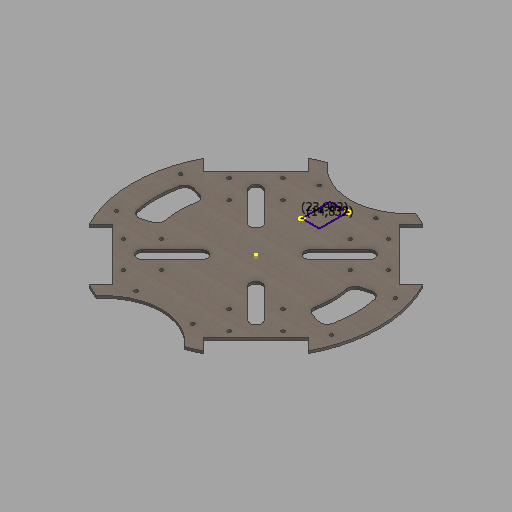
# Autodesk Inventor part: floor_v2
Saved by Autodesk Inventor 2023 (Build 270158000, 158)
## iProperties
Created: 2024-09-07
Part Number: floor_v2
Material: Алюминий 6061
Document SubType Name: Modeling
Designer: Ivan
Density: 2.7 g/cm^3
Appearance: Орех
Mass: 136.784 g
Surface Area: 534.847 cm^2
Volume: 50.6608 cm^3
Author: Ivan
Autodesk Inventor part; units mm, degrees
ref_plane "YZ Plane" through (0, 0, 0) normal (1, 0, 0) x (0, 1, 0)
ref_plane "XZ Plane" through (0, 0, 0) normal (0, 1, 0) x (-1, 0, 0)
ref_plane "XY Plane" through (0, 0, 0) normal (0, 0, 1) x (1, 0, 0)
sketch "Эскиз2" plane through (0, 0, 0) normal (0, 1, 0) x (1, 0, 0)
  circle A0 centre (0, 0) radius 107.5
  circle A1 centre (0, 0) radius 104
  line L0 (0, 0) -> (104, 0) construction
  line L1 (0, 0) -> (0, -104) construction
  line L2 (0, 0) -> (-104, 0) construction
  line L3 (0, 0) -> (0, 104) construction
  line L4 (104, 0) -> (0, -104) construction
  line L5 (0, 104) -> (-104, 0) construction
  line L6 (0, -104) -> (-104, 0) construction
  line L7 (104, 0) -> (0, 104) construction
  line L8 (0, 0) -> (-73.5391, -73.5391) construction
  line L9 (0, 0) -> (73.5391, -73.5391) construction
  line L10 (0, 0) -> (73.5391, 73.5391) construction
  line L11 (0, 0) -> (-73.5391, 73.5391) construction
  line L12 (-38.4471, -82.2877) -> (-82.2877, -38.4471)
  line L13 (-38.4471, -82.2877) -> (-48.2758, -92.1165)
  line L14 (-82.2877, -38.4471) -> (-92.1165, -48.2758)
  line L15 (92.1165, -48.2758) -> (82.2877, -38.4471)
  line L16 (82.2877, -38.4471) -> (38.4471, -82.2877)
  line L17 (38.4471, -82.2877) -> (48.2758, -92.1165)
  line L18 (48.2758, 92.1165) -> (38.4471, 82.2877)
  line L19 (38.4471, 82.2877) -> (82.2877, 38.4471)
  line L20 (82.2877, 38.4471) -> (92.1165, 48.2758)
  line L21 (-48.2758, 92.1165) -> (-38.4471, 82.2877)
  line L22 (-38.4471, 82.2877) -> (-82.2877, 38.4471)
  line L23 (-82.2877, 38.4471) -> (-92.1165, 48.2758)
  line L24 (0, -107.5) -> (0, -79.5) construction
  circle A2 centre (0, -116.5) radius 37 construction
  circle A3 centre (0, -127) radius 47.5
  line L25 (0, 107.5) -> (0, 79.5) construction
  circle A4 centre (0, 127) radius 47.5
  line L26 (-92.1165, 48.2758) -> (-94.7051, 50.8645)
  line L27 (-48.2758, 92.1165) -> (-50.8645, 94.7051)
  line L28 (48.2758, 92.1165) -> (50.8645, 94.7051)
  line L29 (92.1165, 48.2758) -> (94.7051, 50.8645)
  line L30 (92.1165, -48.2758) -> (94.7051, -50.8645)
  line L31 (48.2758, -92.1165) -> (50.8645, -94.7051)
  line L32 (-92.1165, -48.2758) -> (-94.7051, -50.8645)
  line L33 (-48.2758, -92.1165) -> (-50.8645, -94.7051)
  point P0 (-52, -52)
  point P1 (-52, 52)
  point P2 (52, 52)
  point P3 (52, -52)
  point P4 (-60.3674, -60.3674)
  point P5 (60.3674, -60.3674)
  point P6 (60.3674, 60.3674)
  point P7 (-60.3674, 60.3674)
  point P8 (-36.9892, -97.1998)
  point P9 (36.9892, -97.1998)
  point P10 (36.9892, 97.1998)
  point P11 (-36.9892, 97.1998)
  dimension "d137" = 215
  dimension "d138" = 208
  dimension "d143" = 74
  dimension "d144" = 95
  dimension "d140" = 62
  dimension "d141" = 13.9
  dimension "d142" = 28
  constraints: 68 end point, 15 point on line, 14 equal length, 10 perpendicular, 8 collinear, 8 midpoint, 5 parallel, 2 coincident, 2 horizontal, 2 vertical, 1 vertical alignment, 32 other
  measures "d140" distance from line of L14 L12.start
  measures "d141" distance from line of L12 L13.end
  measures "d142" distance of L24.start L24.end
extrude "Выдавливание1" add sketch "Эскиз2" along normal blind 2 contours A1 L15 L16 L17 A3 L13 L12 L14 L23 L22 L21 A4 L18 L19 L20
sketch "Эскиз3" plane through (0, 2, 0) normal (0, -1, 0) x (-1, 0, 0)
  line L0 (33.8509, 77.6915) -> (77.6915, 33.8509) construction
  line L1 (55.7712, 55.7712) -> (0, 0) construction
  line L2 (44.4575, 67.0849) -> (67.0849, 44.4575) construction
  circle A0 centre (44.4575, 67.0849) radius 1.5
  circle A1 centre (67.0849, 44.4575) radius 1.5
  line L3 (28.3991, 51.0265) -> (51.0265, 28.3991) construction
  circle A2 centre (28.3991, 51.0265) radius 1.5
  circle A3 centre (51.0265, 28.3991) radius 1.5
  line L4 (44.4575, -67.0849) -> (67.0849, -44.4575) construction
  line L5 (28.3991, -51.0265) -> (51.0265, -28.3991) construction
  line L6 (55.7712, -55.7712) -> (0, 0) construction
  line L7 (-44.4575, -67.0849) -> (-67.0849, -44.4575) construction
  line L8 (-28.3991, -51.0265) -> (-51.0265, -28.3991) construction
  line L9 (-55.7712, -55.7712) -> (0, 0) construction
  line L10 (-67.0849, 44.4575) -> (-44.4575, 67.0849) construction
  line L11 (-51.0265, 28.3991) -> (-28.3991, 51.0265) construction
  line L12 (-55.7712, 55.7712) -> (0, 0) construction
  circle A4 centre (-44.4575, 67.0849) radius 1.5
  circle A5 centre (-67.0849, 44.4575) radius 1.5
  circle A6 centre (-28.3991, 51.0265) radius 1.5
  circle A7 centre (-51.0265, 28.3991) radius 1.5
  circle A8 centre (-44.4575, -67.0849) radius 1.5
  circle A9 centre (-67.0849, -44.4575) radius 1.5
  circle A10 centre (-51.0265, -28.3991) radius 1.5
  circle A11 centre (-28.3991, -51.0265) radius 1.5
  circle A12 centre (44.4575, -67.0849) radius 1.5
  circle A13 centre (28.3991, -51.0265) radius 1.5
  circle A14 centre (51.0265, -28.3991) radius 1.5
  circle A15 centre (67.0849, -44.4575) radius 1.5
  line L13 (-38.4471, -82.2877) -> (-82.2877, -38.4471) projected
  line L14 (82.2877, -38.4471) -> (38.4471, -82.2877) projected
  line L15 (38.4471, 82.2877) -> (82.2877, 38.4471) projected
  line L16 (-82.2877, 38.4471) -> (-38.4471, 82.2877) projected
  line L17 (82.2877, 38.4471) -> (92.1165, 48.2758) projected
  point P0 (39.7128, 39.7128)
  point P1 (-39.7128, -39.7128)
  point P2 (39.7128, -39.7128)
  point P3 (-39.7128, 39.7128)
  point P4 (-40.1306, -40.1306)
  dimension "d83" = 16
  dimension "d84" = 3
  dimension "d85" = 3
  dimension "d86" = 22.71
  dimension "d87" = 3
  dimension "d88" = 3
  dimension "d89" = 22.71
  dimension "d90" = 22.71
  dimension "d91" = 22.71
  dimension "d95" = 3
  dimension "d96" = 3
  dimension "d97" = 3
  dimension "d98" = 3
  dimension "d99" = 3
  dimension "d100" = 3
  dimension "d101" = 3
  dimension "d102" = 3
  dimension "d103" = 3
  dimension "d104" = 3
  dimension "d105" = 3
  dimension "d106" = 3
  dimension "d145" = 6.5
  dimension "d146" = 6.5
  dimension "d147" = 6.5
  dimension "d148" = 6.5
  constraints: 26 end point, 16 centre point, 16 coincident, 10 point on line, 9 midpoint, 8 equal length, 8 parallel, 2 perpendicular, 1 collinear
  measures "d83" distance from line of L1 L2.start
  measures "d84" diameter of A0
  measures "d85" diameter of A1
  measures "d86" distance from line of L3 L1.start
  measures "d87" diameter of A2
  measures "d88" diameter of A3
  measures "d89" distance from line of L5 L6.start
  measures "d90" distance from line of L11 L12.start
  measures "d91" distance from line of L8 L9.start
  measures "d95" diameter of A4
  measures "d96" diameter of A5
  measures "d97" diameter of A6
  measures "d98" diameter of A7
  measures "d99" diameter of A8
  measures "d100" diameter of A9
  measures "d101" diameter of A10
  measures "d102" diameter of A11
  measures "d103" diameter of A12
  measures "d104" diameter of A13
  measures "d105" diameter of A14
  measures "d106" diameter of A15
  measures "d145" distance from line of L15 L1.start
  measures "d146" distance from line of L16 L12.start
  measures "d147" distance from line of L13 L9.start
  measures "d148" distance from line of L6.start L14
extrude "Выдавливание5" cut sketch "Эскиз3" along normal through all
sketch "Эскиз6" plane through (0, 2, 0) normal (0, -1, 0) x (-1, 0, 0)
  arc A0 (36.9892, -97.1998) -> (-36.9892, -97.1998) centre (0, -127) ccw projected
  arc A1 (-36.9892, 97.1998) -> (36.9892, 97.1998) centre (0, 127) ccw projected
  point P0 (-0.0301, 154.5629)
  point P1 (-0.0412, -154.5628)
sketch "Эскиз7" plane through (0, 2, 0) normal (0, -1, 0) x (-1, 0, 0)
  circle A0 centre (0, 0) radius 94.2655 construction
  circle A1 centre (-90.3481, 26.8924) radius 1.5
  circle A2 centre (-90.3481, -26.8924) radius 1.5
  circle A3 centre (90.3481, 26.8924) radius 1.5
  circle A4 centre (90.3481, -26.8924) radius 1.5
  line L0 (-92.1165, 48.2758) -> (-82.2877, 38.4471) projected
  line L1 (-82.2877, -38.4471) -> (-92.1165, -48.2758) projected
  line L2 (92.1165, -48.2758) -> (82.2877, -38.4471) projected
  line L3 (82.2877, 38.4471) -> (92.1165, 48.2758) projected
  dimension "d119" = 188.531
  dimension "d120" = 3
  dimension "d121" = 3
  dimension "d124" = 3
  dimension "d125" = 3
  dimension "d149" = 13.87
  dimension "d150" = 13.87
  dimension "d151" = 13.87
  dimension "d152" = 13.87
  constraints: 5 centre point, 4 point on circle, 1 coincident
  measures "d119" diameter of A0
  measures "d120" diameter of A1
  measures "d121" diameter of A2
  measures "d124" diameter of A3
  measures "d125" diameter of A4
  measures "d149" distance from line of L0 A1.centre
  measures "d150" distance from line of L1 A2.centre
  measures "d151" distance from line of L2 A4.centre
  measures "d152" distance from line of L3 A3.centre
extrude "Выдавливание4" cut sketch "Эскиз7" along normal through all
sketch "Эскиз8" plane through (0, 2, 0) normal (0, 1, 0) x (1, 0, 0)
  arc A0 (-48.2758, -92.1165) -> (-36.9892, -97.1998) centre (0, 0) ccw projected
  arc A1 (36.9892, -97.1998) -> (48.2758, -92.1165) centre (0, 0) ccw projected
  arc A2 (36.9892, -97.1998) -> (-36.9892, -97.1998) centre (0, -127) ccw projected
  circle A3 centre (0, -127) radius 55.4164 construction
  circle A4 centre (-23.8556, -76.9811) radius 1.5
  circle A5 centre (23.8556, -76.9811) radius 1.5
  circle A6 centre (-28.3991, -51.0265) radius 1.5 construction
  circle A7 centre (-51.0265, -28.3991) radius 1.5 construction
  circle A8 centre (-67.0849, -44.4575) radius 1.5 construction
  circle A9 centre (-44.4575, -67.0849) radius 1.5 construction
  circle A10 centre (-51.0265, -28.3991) radius 1.5 construction
  line L0 (-51.0265, -28.3991) -> (-28.3991, -51.0265) construction
  line L1 (-67.0849, -44.4575) -> (-44.4575, -67.0849) construction
  line L2 (-55.7712, -55.7712) -> (-39.7128, -39.7128) construction
  line L3 (-50.4184, -50.4184) -> (-23.8556, -76.9811) construction
  circle A11 centre (67.0849, -44.4575) radius 1.5 construction
  circle A12 centre (44.4575, -67.0849) radius 1.5 construction
  line L4 (44.4575, -67.0849) -> (67.0849, -44.4575) construction
  arc A13 (-92.1165, 48.2758) -> (-92.1165, -48.2758) centre (0, 0) ccw construction
  line L5 (-104, 0) -> (104, 0) construction
  arc A14 (92.1165, -48.2758) -> (92.1165, 48.2758) centre (0, 0) ccw construction
  circle A15 centre (-23.8556, 76.9811) radius 1.5
  circle A16 centre (23.8556, 76.9811) radius 1.5
  point P0 (-44.5136, -93.9922)
  point P1 (-104, 0)
  dimension "d153" = 11.2867
  dimension "d154" = 3.7622
  dimension "d156" = 22.71
  dimension "d157" = 7.57
  dimension "d158" = 7.57
  constraints: 12 end point, 7 point on circle, 5 centre point, 2 equal radius, 2 midpoint, 2 symmetric about line, 1 coincident, 1 horizontal, 1 perpendicular, 1 point on line, 2 other
  measures "d153" horizontal distance of A0.end A0.start
  measures "d154" horizontal distance of A3.start A0.start
  measures "d156" distance from line of L0 L2.start
  measures "d157" distance from line of L1 L3.start
  measures "d158" distance from line of L4 A5.centre
extrude "Выдавливание6" cut sketch "Эскиз8" against normal through all
sketch "Эскиз9" plane through (0, 2, 0) normal (0, 1, 0) x (1, 0, 0)
  circle A0 centre (-23.8556, 76.9811) radius 1.5 projected
  circle A1 centre (23.8556, -76.9811) radius 1.5 projected
  circle A2 centre (23.8556, 76.9811) radius 1.5 projected
  circle A3 centre (-23.8556, -76.9811) radius 1.5 projected
  circle A4 centre (-90.3481, 26.8924) radius 1.5 projected
  circle A5 centre (90.3481, -26.8924) radius 1.5 projected
  circle A6 centre (-90.3481, -26.8924) radius 1.5 projected
  circle A7 centre (90.3481, 26.8924) radius 1.5 projected
  circle A8 centre (51.0265, -28.3991) radius 1.5 projected
  circle A9 centre (-67.0849, -44.4575) radius 1.5 projected
  circle A10 centre (-44.4575, 67.0849) radius 1.5 projected
  circle A11 centre (51.0265, 28.3991) radius 1.5 projected
  circle A12 centre (28.3991, 51.0265) radius 1.5 projected
  circle A13 centre (-67.0849, 44.4575) radius 1.5 projected
  circle A14 centre (-28.3991, -51.0265) radius 1.5 projected
  circle A15 centre (28.3991, -51.0265) radius 1.5 projected
  circle A16 centre (67.0849, -44.4575) radius 1.5 projected
  circle A17 centre (-51.0265, -28.3991) radius 1.5 projected
  circle A18 centre (-28.3991, 51.0265) radius 1.5 projected
  circle A19 centre (67.0849, 44.4575) radius 1.5 projected
  circle A20 centre (44.4575, 67.0849) radius 1.5 projected
  circle A21 centre (-51.0265, 28.3991) radius 1.5 projected
  circle A22 centre (-44.4575, -67.0849) radius 1.5 projected
  circle A23 centre (44.4575, -67.0849) radius 1.5 projected
  line L0 (-82.2877, 38.4471) -> (-92.1165, 48.2758) projected
  arc A24 (-92.1165, 48.2758) -> (-92.1165, -48.2758) centre (0, 0) ccw projected
  line L1 (-92.1165, -48.2758) -> (-82.2877, -38.4471) projected
  line L2 (-82.2877, -38.4471) -> (-38.4471, -82.2877) projected
  line L3 (-38.4471, -82.2877) -> (-48.2758, -92.1165) projected
  arc A25 (-48.2758, -92.1165) -> (-36.9892, -97.1998) centre (0, 0) ccw projected
  arc A26 (36.9892, -97.1998) -> (-36.9892, -97.1998) centre (0, -127) ccw projected
  arc A27 (36.9892, -97.1998) -> (48.2758, -92.1165) centre (0, 0) ccw projected
  line L4 (48.2758, -92.1165) -> (38.4471, -82.2877) projected
  line L5 (38.4471, -82.2877) -> (82.2877, -38.4471) projected
  line L6 (82.2877, -38.4471) -> (92.1165, -48.2758) projected
  arc A28 (92.1165, -48.2758) -> (92.1165, 48.2758) centre (0, 0) ccw projected
  line L7 (92.1165, 48.2758) -> (82.2877, 38.4471) projected
  line L8 (82.2877, 38.4471) -> (38.4471, 82.2877) projected
  line L9 (38.4471, 82.2877) -> (48.2758, 92.1165) projected
  arc A29 (48.2758, 92.1165) -> (36.9892, 97.1998) centre (0, 0) ccw projected
  arc A30 (-36.9892, 97.1998) -> (36.9892, 97.1998) centre (0, 127) ccw projected
  arc A31 (-36.9892, 97.1998) -> (-48.2758, 92.1165) centre (0, 0) ccw projected
  line L10 (-48.2758, 92.1165) -> (-38.4471, 82.2877) projected
  line L11 (-38.4471, 82.2877) -> (-82.2877, 38.4471) projected
  circle A32 centre (-51.0265, 28.3991) radius 1.5 projected
  circle A33 centre (-51.0265, 28.3991) radius 6
  circle A34 centre (-28.3991, 51.0265) radius 1.5 projected
  circle A35 centre (-28.3991, 51.0265) radius 6
  line L12 (-55.2691, 32.6417) -> (-46.7838, 24.1564) construction
  line L13 (-32.6417, 55.2691) -> (-24.1564, 46.7838) construction
  line L14 (-38.4471, 82.2877) -> (-82.2877, 38.4471) projected
  line L15 (-24.1564, 46.7838) -> (-46.7838, 24.1564)
  line L16 (-68.8527, 33.4973) -> (-33.4973, 68.8527)
  line L17 (-55.2691, 32.6417) -> (-32.6417, 55.2691)
  line L18 (-82.2877, 38.4471) -> (-77.3379, 33.4973)
  line L19 (-38.4471, 82.2877) -> (-33.4973, 77.3379)
  line L20 (-51.175, 51.175) -> (-43.9554, 43.9554) construction
  arc A36 (-33.4973, 68.8527) -> (-33.4973, 77.3379) centre (-37.74, 73.0953) ccw
  line L21 (-33.4973, 68.8527) -> (-37.74, 73.0953) construction
  line L22 (-37.74, 73.0953) -> (-33.4973, 77.3379) construction
  arc A37 (-77.3379, 33.4973) -> (-68.8527, 33.4973) centre (-73.0953, 37.74) ccw
  line L23 (-46.7838, -24.1564) -> (-24.1564, -46.7838)
  circle A38 centre (-28.3991, -51.0265) radius 6
  circle A39 centre (-51.0265, -28.3991) radius 6
  line L24 (-32.6417, -55.2691) -> (-55.2691, -32.6417)
  line L25 (-33.4973, -68.8527) -> (-68.8527, -33.4973)
  arc A40 (-68.8527, -33.4973) -> (-77.3379, -33.4973) centre (-73.0953, -37.74) ccw
  line L26 (-82.2877, -38.4471) -> (-77.3379, -33.4973)
  line L27 (-38.4471, -82.2877) -> (-33.4973, -77.3379)
  arc A41 (-33.4973, -77.3379) -> (-33.4973, -68.8527) centre (-37.74, -73.0953) ccw
  line L28 (24.1564, -46.7838) -> (46.7838, -24.1564)
  circle A42 centre (51.0265, -28.3991) radius 6
  circle A43 centre (28.3991, -51.0265) radius 6
  line L29 (55.2691, -32.6417) -> (32.6417, -55.2691)
  line L30 (68.8527, -33.4973) -> (33.4973, -68.8527)
  arc A44 (33.4973, -68.8527) -> (33.4973, -77.3379) centre (37.74, -73.0953) ccw
  line L31 (38.4471, -82.2877) -> (33.4973, -77.3379)
  line L32 (82.2877, -38.4471) -> (77.3379, -33.4973)
  arc A45 (77.3379, -33.4973) -> (68.8527, -33.4973) centre (73.0953, -37.74) ccw
  line L33 (46.7838, 24.1564) -> (24.1564, 46.7838)
  circle A46 centre (28.3991, 51.0265) radius 6
  circle A47 centre (51.0265, 28.3991) radius 6
  line L34 (32.6417, 55.2691) -> (55.2691, 32.6417)
  line L35 (33.4973, 68.8527) -> (68.8527, 33.4973)
  arc A48 (68.8527, 33.4973) -> (77.3379, 33.4973) centre (73.0953, 37.74) ccw
  line L36 (82.2877, 38.4471) -> (77.3379, 33.4973)
  line L37 (38.4471, 82.2877) -> (33.4973, 77.3379)
  arc A49 (33.4973, 77.3379) -> (33.4973, 68.8527) centre (37.74, 73.0953) ccw
  point P0 (-43.9554, -43.9554)
  point P1 (-51.175, -51.175)
  point P2 (43.9554, -43.9554)
  point P3 (51.175, -51.175)
  point P4 (43.9554, 43.9554)
  point P5 (51.175, 51.175)
  dimension "d161" = 12
  dimension "d162" = 10.21
  dimension "d163" = 7
  dimension "d164" = 6
  dimension "d167" = 360
  constraints: 50 end point, 32 point on circle, 16 centre point, 7 perpendicular, 5 coincident, 4 midpoint, 2 equal radius, 2 parallel, 101 other
  measures "d161" diameter of A33
  measures "d162" distance between parallel lines of L16 L17
  measures "d163" distance from line of L11 L19.end
  measures "d164" radius of A36
sketch "Эскиз10" plane through (0, 2, 0) normal (0, 1, 0) x (1, 0, 0)
  circle A0 centre (-23.8556, 76.9811) radius 1.5 projected
  circle A1 centre (23.8556, -76.9811) radius 1.5 projected
  circle A2 centre (23.8556, 76.9811) radius 1.5 projected
  circle A3 centre (-23.8556, -76.9811) radius 1.5 projected
  circle A4 centre (-90.3481, 26.8924) radius 1.5 projected
  circle A5 centre (90.3481, -26.8924) radius 1.5 projected
  circle A6 centre (-90.3481, -26.8924) radius 1.5 projected
  circle A7 centre (90.3481, 26.8924) radius 1.5 projected
  circle A8 centre (51.0265, -28.3991) radius 1.5 projected
  circle A9 centre (-67.0849, -44.4575) radius 1.5 projected
  circle A10 centre (-44.4575, 67.0849) radius 1.5 projected
  circle A11 centre (51.0265, 28.3991) radius 1.5 projected
  circle A12 centre (28.3991, 51.0265) radius 1.5 projected
  circle A13 centre (-67.0849, 44.4575) radius 1.5 projected
  circle A14 centre (-28.3991, -51.0265) radius 1.5 projected
  circle A15 centre (28.3991, -51.0265) radius 1.5 projected
  circle A16 centre (67.0849, -44.4575) radius 1.5 projected
  circle A17 centre (-51.0265, -28.3991) radius 1.5 projected
  circle A18 centre (-28.3991, 51.0265) radius 1.5 projected
  circle A19 centre (67.0849, 44.4575) radius 1.5 projected
  circle A20 centre (44.4575, 67.0849) radius 1.5 projected
  circle A21 centre (-51.0265, 28.3991) radius 1.5 projected
  circle A22 centre (-44.4575, -67.0849) radius 1.5 projected
  circle A23 centre (44.4575, -67.0849) radius 1.5 projected
  line L0 (-82.2877, 38.4471) -> (-92.1165, 48.2758) projected
  arc A24 (-92.1165, 48.2758) -> (-92.1165, -48.2758) centre (0, 0) ccw projected
  line L1 (-92.1165, -48.2758) -> (-82.2877, -38.4471) projected
  line L2 (-82.2877, -38.4471) -> (-38.4471, -82.2877) projected
  line L3 (-38.4471, -82.2877) -> (-48.2758, -92.1165) projected
  arc A25 (-48.2758, -92.1165) -> (-36.9892, -97.1998) centre (0, 0) ccw projected
  arc A26 (36.9892, -97.1998) -> (-36.9892, -97.1998) centre (0, -127) ccw projected
  arc A27 (36.9892, -97.1998) -> (48.2758, -92.1165) centre (0, 0) ccw projected
  line L4 (48.2758, -92.1165) -> (38.4471, -82.2877) projected
  line L5 (38.4471, -82.2877) -> (82.2877, -38.4471) projected
  line L6 (82.2877, -38.4471) -> (92.1165, -48.2758) projected
  arc A28 (92.1165, -48.2758) -> (92.1165, 48.2758) centre (0, 0) ccw projected
  line L7 (92.1165, 48.2758) -> (82.2877, 38.4471) projected
  line L8 (82.2877, 38.4471) -> (38.4471, 82.2877) projected
  line L9 (38.4471, 82.2877) -> (48.2758, 92.1165) projected
  arc A29 (48.2758, 92.1165) -> (36.9892, 97.1998) centre (0, 0) ccw projected
  arc A30 (-36.9892, 97.1998) -> (36.9892, 97.1998) centre (0, 127) ccw projected
  arc A31 (-36.9892, 97.1998) -> (-48.2758, 92.1165) centre (0, 0) ccw projected
  line L10 (-48.2758, 92.1165) -> (-38.4471, 82.2877) projected
  line L11 (-38.4471, 82.2877) -> (-82.2877, 38.4471) projected
  line L12 (-68.8527, 33.4973) -> (-33.4973, 68.8527) projected
  line L13 (-51.175, 51.175) -> (-43.9554, 43.9554) construction
  line L14 (-55.2691, 32.6417) -> (-32.6417, 55.2691) projected
  circle A32 centre (-47.5652, 47.5652) radius 5.105
  line L15 (-51.175, 43.9554) -> (-43.9554, 51.175) construction
  line L16 (-51.175, 43.9554) -> (-26.5747, 19.3552)
  line L17 (-43.9554, 51.175) -> (-19.3552, 26.5747)
  line L18 (-26.5747, 19.3552) -> (-19.3552, 26.5747) construction
  arc A33 (-26.5747, 19.3552) -> (-19.3552, 26.5747) centre (-22.965, 22.965) ccw
  circle A34 centre (-47.5652, -47.5652) radius 5.105
  line L19 (-51.175, -43.9554) -> (-26.5747, -19.3552)
  line L20 (-43.9554, -51.175) -> (-19.3552, -26.5747)
  arc A35 (-19.3552, -26.5747) -> (-26.5747, -19.3552) centre (-22.965, -22.965) ccw
  circle A36 centre (47.5652, -47.5652) radius 5.105
  line L21 (43.9554, -51.175) -> (19.3552, -26.5747)
  line L22 (51.175, -43.9554) -> (26.5747, -19.3552)
  arc A37 (26.5747, -19.3552) -> (19.3552, -26.5747) centre (22.965, -22.965) ccw
  circle A38 centre (47.5652, 47.5652) radius 5.105
  line L23 (51.175, 43.9554) -> (26.5747, 19.3552)
  line L24 (43.9554, 51.175) -> (19.3552, 26.5747)
  arc A39 (19.3552, 26.5747) -> (26.5747, 19.3552) centre (22.965, 22.965) ccw
  point P0 (-19.3552, 19.3552)
  point P1 (-51.175, -51.175)
  point P2 (-19.3552, -19.3552)
  point P3 (51.175, -51.175)
  point P4 (19.3552, -19.3552)
  point P5 (51.175, 51.175)
  point P6 (19.3552, 19.3552)
  dimension "d169" = 45
  dimension "d172" = 360
  constraints: 24 point on circle, 20 end point, 8 centre point, 3 midpoint, 2 parallel, 2 perpendicular, 1 coincident, 1 point on line, 49 other
  measures "d169" distance from line of L12 point (-19.355, 19.355)
extrude "Выдавливание7" cut sketch "Эскиз10" against normal through all contours L16 A32 L14 | L14 L17 A33 L16 | A32 L17 L14 | A32 | A34 | A34 L19 A35 L20 | A36 | A36 L21 A37 L22 | A38 | A38 L23 A39 L24
sketch "Эскиз12" plane through (0, 2, 0) normal (0, 1, 0) x (1, 0, 0)
  circle A0 centre (0, 0) radius 64.397
  circle A1 centre (-51.0265, 28.3991) radius 6 projected
  arc A2 (-77.3379, 33.4973) -> (-68.8527, 33.4973) centre (-73.0953, 37.74) ccw projected
  circle A3 centre (0, 0) radius 84.2806
  circle A4 centre (-90.3481, 26.8924) radius 1.5 projected
  line L0 (-90.3481, 26.8924) -> (0, 0)
  circle A5 centre (-90.3481, -26.8924) radius 1.5 projected
  line L1 (0, 0) -> (-90.3481, -26.8924)
  point P0 (-80.7782, -24.0439)
  point P1 (-61.7209, -18.3714)
  point P2 (-61.7209, 18.3714)
  point P3 (-80.7782, 24.0439)
  constraints: 5 coincident, 4 end point, 1 centre point, 1 tangent, 3 other
extrude "Выдавливание10" cut sketch "Эскиз12" against normal up to surface (2 mm away) contours L1 A3 L0 A0 picked at (-77.3593, -4.0496)
fillet "Сопряжение3" radius 6 4 edges at (-61.7209, 1, 18.3714) (-80.7782, 1, 24.0439) (-61.7209, 1, -18.3714) (-80.7782, 1, -24.0439)
mirror "Зеркальное отражение1" about plane through (0, 0, 0) normal (1, 0, 0) of "Сопряжение3", "Выдавливание10"
sketch "Эскиз13" plane through (0, 0, 0) normal (0, -1, 0) x (1, 0, 0)
  point P0 (0, 0)
sketch "Эскиз14" plane through (0, 2, 0) normal (0, 1, 0) x (1, 0, 0)
  circle A0 centre (-7.588, 45.6822) radius 2 projected
  circle A1 centre (7.2444, 69.6638) radius 2 projected
  line L0 (7.2444, 69.6638) -> (-7.588, 69.6638)
  line L1 (-7.588, 69.6638) -> (-7.588, 45.6822)
  line L2 (-7.588, 45.6822) -> (7.2444, 45.6822)
  line L3 (7.2444, 45.6822) -> (7.2444, 69.6638)
  point P0 (0, 0)
  dimension "d185" = 23.9816
  dimension "d186" = 14.8324
  constraints: 8 end point, 2 parallel, 1 horizontal, 1 perpendicular
  measures "d185" distance of L0.end L1.end
  measures "d186" distance of L0.start L0.end
equation "\"d85\" = d84"
equation "\"d87\" = d84"
equation "\"d88\" = d84"
